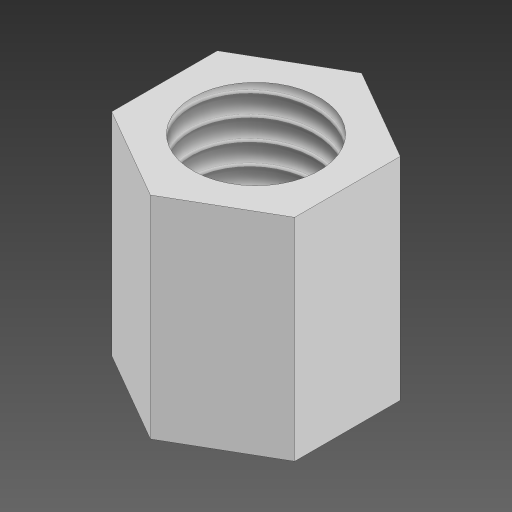
# Autodesk Inventor part: rack_25
Saved by Autodesk Inventor 2023 (Build 270158000, 158)
## iProperties
Created: 2025-07-14
Part Number: rack_25
Material: Типовые
Document SubType Name: Modeling
Designer: daa
Density: 1 g/cm^3
Appearance: По умолчанию
Author: daa
Autodesk Inventor part; units mm, degrees
ref_plane "YZ Plane" through (0, 0, 0) normal (1, 0, 0) x (0, 1, 0)
ref_plane "XZ Plane" through (0, 0, 0) normal (0, 1, 0) x (-1, 0, 0)
ref_plane "XY Plane" through (0, 0, 0) normal (0, 0, 1) x (1, 0, 0)
sketch "Эскиз1" plane through (0, 0, 0) normal (0, 1, 0) x (-1, 0, 0)
  line L0 (0, 0) -> (0, 5)
  line L1 (0, 0) -> (-2.1651, 1.25)
  line L2 (-2.1651, 1.25) -> (-2.1651, 3.75)
  line L3 (-2.1651, 3.75) -> (0, 5)
  line L4 (0, 5) -> (2.1651, 3.75)
  line L5 (2.1651, 3.75) -> (2.1651, 1.25)
  line L6 (2.1651, 1.25) -> (0, 0)
  circle A0 centre (0, 2.5) radius 1.5
  dimension "d0" = 5
  dimension "d1" = 3
  constraints: 14 end point, 1 centre point, 1 coincident, 1 midpoint, 1 vertical, 13 other
  measures "d0" distance of L0.start L0.end
  measures "d1" diameter of A0
extrude "Выдавливание1" add sketch "Эскиз1" along normal blind 5 contours L1 L2 L3 L0 A0 | L0 A0 L4 L5 L6
thread "Резьба1" size "M3x0.5" class "6H" standard "ANSI Metric M Profile" full length
